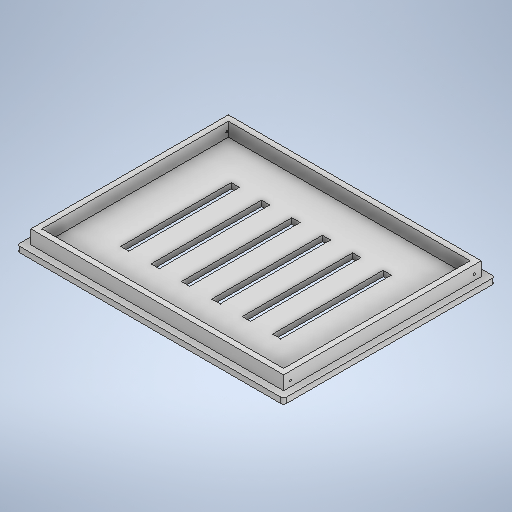
# Autodesk Inventor part: Kondensatorbox
Saved by Autodesk Inventor 2025 (Build 290162010, 162A)
## iProperties
Created: 2024-10-11
Part Number: Kondensatorbox
Material: Generisch
Document SubType Name: Modeling
Designer: max-h
Density: 1 g/cm^3
Appearance: Vorgabe
Author: max-h
Autodesk Inventor part; units mm, degrees
ref_plane "YZ Plane" through (0, 0, 0) normal (1, 0, 0) x (0, 1, 0)
ref_plane "XZ Plane" through (0, 0, 0) normal (0, 1, 0) x (-1, 0, 0)
ref_plane "XY Plane" through (0, 0, 0) normal (0, 0, 1) x (1, 0, 0)
sketch "Skizze1" plane through (0, 0, 0) normal (0, 1, 0) x (-1, 0, 0)
  line L0 (90.5, 0) -> (0, 0) construction
  line L1 (0, 0) -> (0, -70.5) construction
  line L2 (0, -70.5) -> (90.5, -70.5) construction
  line L3 (90.5, -70.5) -> (90.5, 0) construction
  line L4 (93.5, 3) -> (-3, 3)
  line L5 (-3, 3) -> (-3, -73.5)
  line L6 (-3, -73.5) -> (93.5, -73.5)
  line L7 (93.5, -73.5) -> (93.5, 3)
  dimension "d0" = 70.5
  dimension "d1" = 90.5
  dimension "d2" = 3
  dimension "d3" = 3
  dimension "d4" = 3
  dimension "d5" = 3
  constraints: 16 end point, 4 parallel, 2 horizontal, 2 perpendicular, 1 coincident
  measures "d0" distance of L2.end L0.start
  measures "d1" distance of L1.end L2.end
  measures "d2" distance between parallel lines of L7 L3
  measures "d3" distance between parallel lines of L4 L0
  measures "d4" distance between parallel lines of L5 L1
  measures "d5" distance between parallel lines of L6 L2
extrude "Extrusion1" add sketch "Skizze1" along normal blind 2
sketch "Skizze7" plane through (0, 2, 0) normal (0, 1, 0) x (1, 0, 0)
  line L0 (-91, -0.5) -> (0.5, -0.5)
  line L1 (0.5, -0.5) -> (0.5, 71)
  line L2 (0.5, 71) -> (-91, 71)
  line L3 (-91, 71) -> (-91, -0.5)
  line L4 (3, -3) -> (3, 73.5) projected
  line L5 (-93.5, -3) -> (3, -3) projected
  line L6 (3, 73.5) -> (-93.5, 73.5) projected
  line L7 (-93.5, 73.5) -> (-93.5, -3) projected
  line L8 (-89, 1.5) -> (-1.5, 1.5)
  line L9 (-1.5, 1.5) -> (-1.5, 69)
  line L10 (-1.5, 69) -> (-89, 69)
  line L11 (-89, 69) -> (-89, 1.5)
  point P0 (0, 0)
  dimension "d51" = 2.5
  dimension "d52" = 2.5
  dimension "d53" = 2.5
  dimension "d54" = 2.5
  dimension "d55" = 2
  dimension "d56" = 2
  dimension "d57" = 2
  dimension "d58" = 2
  constraints: 16 end point, 4 parallel, 2 horizontal, 2 perpendicular
  measures "d51" distance between parallel lines of L4 L1
  measures "d52" distance between parallel lines of L5 L0
  measures "d53" distance between parallel lines of L6 L2
  measures "d54" distance between parallel lines of L7 L3
  measures "d55" distance between parallel lines of L3 L11
  measures "d56" distance between parallel lines of L2 L10
  measures "d57" distance between parallel lines of L1 L9
  measures "d58" distance between parallel lines of L0 L8
extrude "Extrusion7" add sketch "Skizze7" along normal blind 5 contours L3 L2 L1 L0
sketch "Skizze8" plane through (0.5, 2, 0.5) normal (1, 0, 0) x (0, 0, -1)
  circle A0 centre (2.5, 2) radius 0.4
  circle A1 centre (69, 2) radius 0.4
  line L0 (-2.5, 0) -> (74, 0) projected
  line L1 (74, -2) -> (74, 0) projected
  line L2 (-2.5, -2) -> (-2.5, 0) projected
  point P0 (0.5, -2)
  dimension "d61" = 2
  dimension "d62" = 5
  dimension "d63" = 2
  dimension "d64" = 5
  dimension "d65" = 0.8
  constraints: 2 centre point, 1 equal radius
  measures "d61" distance from line of L0 A1.centre
  measures "d62" distance from line of L1 A1.centre
  measures "d63" distance from line of L0 A0.centre
  measures "d64" distance from line of L2 A0.centre
  measures "d65" diameter of A0
extrude "Extrusion8" cut sketch "Skizze8" against normal through all
fillet "Rundung2" radius 1 4 edges at (3, 1, 3) (3, 1, -73.5) (-93.5, 1, -73.5) (-93.5, 1, 3)
sketch "Skizze9" plane through (0, 2, 0) normal (0, 1, 0) x (1, 0, 0)
  line L0 (-19.25, 15.25) -> (-16.25, 15.25)
  line L1 (-16.25, 15.25) -> (-16.25, 55.25)
  line L2 (-16.25, 55.25) -> (-19.25, 55.25)
  line L3 (-19.25, 55.25) -> (-19.25, 15.25)
  line L4 (-30.25, 15.25) -> (-27.25, 15.25)
  line L5 (-27.25, 15.25) -> (-27.25, 55.25)
  line L6 (-27.25, 55.25) -> (-30.25, 55.25)
  line L7 (-30.25, 55.25) -> (-30.25, 15.25)
  line L8 (-41.25, 15.25) -> (-38.25, 15.25)
  line L9 (-38.25, 15.25) -> (-38.25, 55.25)
  line L10 (-38.25, 55.25) -> (-41.25, 55.25)
  line L11 (-41.25, 55.25) -> (-41.25, 15.25)
  line L12 (-52.25, 15.25) -> (-49.25, 15.25)
  line L13 (-49.25, 15.25) -> (-49.25, 55.25)
  line L14 (-49.25, 55.25) -> (-52.25, 55.25)
  line L15 (-52.25, 55.25) -> (-52.25, 15.25)
  line L16 (-89, 1.5) -> (-1.5, 1.5) projected
  line L17 (-1.5, 1.5) -> (-1.5, 69) projected
  line L18 (-63.25, 55.25) -> (-60.25, 55.25)
  line L19 (-60.25, 55.25) -> (-60.25, 15.25)
  line L20 (-60.25, 15.25) -> (-63.25, 15.25)
  line L21 (-63.25, 15.25) -> (-63.25, 55.25)
  line L22 (-74.25, 55.25) -> (-71.25, 55.25)
  line L23 (-71.25, 55.25) -> (-71.25, 15.25)
  line L24 (-71.25, 15.25) -> (-74.25, 15.25)
  line L25 (-74.25, 15.25) -> (-74.25, 55.25)
  point P0 (0, 0)
  point P1 (-49.25, 35.25)
  point P2 (-41.25, 35.25)
  point P3 (-38.25, 35.25)
  dimension "d69" = 3
  dimension "d70" = 8
  dimension "d71" = 8
  dimension "d72" = 8
  dimension "d73" = 40
  dimension "d74" = 13.75
  dimension "d75" = 14.75
  dimension "d78" = 8
  dimension "d79" = 8
  constraints: 48 end point, 12 parallel, 10 equal length, 6 horizontal, 6 perpendicular, 3 midpoint, 3 point on line, 2 collinear
  measures "d69" distance of L12.start L12.end
  measures "d70" distance of point (-49.25, 35.25) point (-41.25, 35.25)
  measures "d71" distance from line of L7 point (-38.25, 35.25)
  measures "d72" distance between parallel lines of L3 L5
  measures "d73" distance of L14.end L12.start
  measures "d74" distance between parallel lines of L16 L12
  measures "d75" distance between parallel lines of L17 L1
  measures "d78" distance between parallel lines of L19 L15
  measures "d79" distance between parallel lines of L23 L21
extrude "Extrusion9" cut sketch "Skizze9" against normal blind 10
